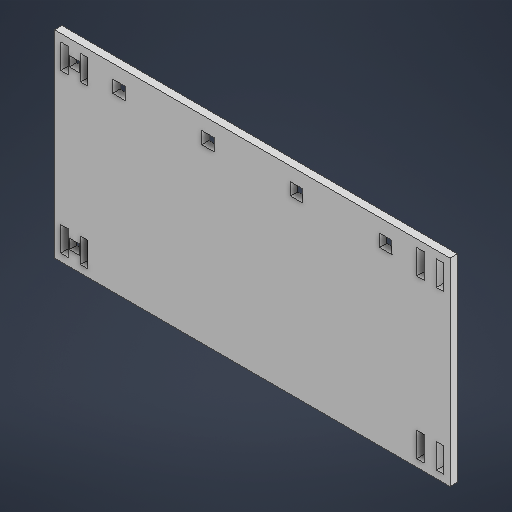
# Autodesk Inventor part: techo
Saved by Autodesk Inventor 2026 (Build 300175000, 175)
## iProperties
Created: 2026-05-15
Part Number: techo
Material: Generic
Document SubType Name: Modeling
Designer: juana
Density: 1 g/cm^3
Appearance: Default
Author: juana
Autodesk Inventor part; units mm, degrees
ref_plane "YZ Plane" through (0, 0, 0) normal (1, 0, 0) x (0, 1, 0)
ref_plane "XZ Plane" through (0, 0, 0) normal (0, 1, 0) x (-1, 0, 0)
ref_plane "XY Plane" through (0, 0, 0) normal (0, 0, 1) x (1, 0, 0)
sketch "Sketch1" plane through (0, 0, 0) normal (0, 0, 1) x (1, 0, 0)
  line L0 (0, 0) -> (160, 0)
  line L1 (160, 0) -> (160, 80)
  line L2 (160, 80) -> (0, 80)
  line L3 (0, 80) -> (0, 0)
  line L4 (2.5, 13) -> (5.5, 13)
  line L5 (5.5, 13) -> (5.5, 3)
  line L6 (5.5, 3) -> (2.5, 3)
  line L7 (2.5, 3) -> (2.5, 13)
  line L8 (10.5, 13) -> (13.5, 13)
  line L9 (13.5, 13) -> (13.5, 3)
  line L10 (13.5, 3) -> (10.5, 3)
  line L11 (10.5, 3) -> (10.5, 13)
  line L12 (0, 40) -> (160, 40) construction
  line L13 (80, 80) -> (80, 0) construction
  line L14 (0, 0) -> (0, 80)
  line L15 (2.5, 67) -> (5.5, 67)
  line L16 (5.5, 67) -> (5.5, 77)
  line L17 (5.5, 77) -> (2.5, 77)
  line L18 (2.5, 77) -> (2.5, 67)
  line L19 (10.5, 67) -> (13.5, 67)
  line L20 (13.5, 67) -> (13.5, 77)
  line L21 (13.5, 77) -> (10.5, 77)
  line L22 (10.5, 77) -> (10.5, 67)
  line L23 (157.5, 13) -> (154.5, 13)
  line L24 (154.5, 13) -> (154.5, 3)
  line L25 (154.5, 3) -> (157.5, 3)
  line L26 (157.5, 3) -> (157.5, 13)
  line L27 (149.5, 13) -> (146.5, 13)
  line L28 (146.5, 13) -> (146.5, 3)
  line L29 (146.5, 3) -> (149.5, 3)
  line L30 (149.5, 3) -> (149.5, 13)
  line L31 (154.5, 67) -> (154.5, 77)
  line L32 (157.5, 67) -> (154.5, 67)
  line L33 (157.5, 77) -> (157.5, 67)
  line L34 (146.5, 77) -> (149.5, 77)
  line L35 (149.5, 77) -> (149.5, 67)
  line L36 (149.5, 67) -> (146.5, 67)
  line L37 (146.5, 67) -> (146.5, 77)
  line L38 (154.5, 77) -> (157.5, 77)
  line L39 (2.5, 77) -> (157.5, 77) construction
  line L40 (157.5, 77) -> (157.5, 3) construction
  line L41 (157.5, 3) -> (2.5, 3) construction
  line L42 (2.5, 3) -> (2.5, 77) construction
  line L43 (6, 74) -> (10, 74)
  line L44 (10, 74) -> (10, 70)
  line L45 (10, 70) -> (6, 70)
  line L46 (6, 70) -> (6, 74)
  line L47 (5.5, 13) -> (5.5, 3)
  line L48 (6, 6) -> (10, 6)
  line L49 (10, 6) -> (10, 10)
  line L50 (10, 10) -> (6, 10)
  line L51 (6, 10) -> (6, 6)
  line L52 (23.49, 69.49) -> (28.51, 69.49)
  line L53 (28.51, 69.49) -> (28.51, 74.51)
  line L54 (28.51, 74.51) -> (23.49, 74.51)
  line L55 (23.49, 74.51) -> (23.49, 69.49)
  line L56 (59.49, 69.49) -> (64.51, 69.49)
  line L57 (64.51, 74.51) -> (59.49, 74.51)
  line L58 (64.51, 69.49) -> (64.51, 74.51)
  line L59 (59.49, 74.51) -> (59.49, 69.49)
  line L60 (95.49, 69.49) -> (100.51, 69.49)
  line L61 (100.51, 74.51) -> (95.49, 74.51)
  line L62 (100.51, 69.49) -> (100.51, 74.51)
  line L63 (95.49, 74.51) -> (95.49, 69.49)
  line L64 (131.49, 69.49) -> (136.51, 69.49)
  line L65 (136.51, 74.51) -> (131.49, 74.51)
  line L66 (136.51, 69.49) -> (136.51, 74.51)
  line L67 (131.49, 74.51) -> (131.49, 69.49)
  point P0 (23.49, 72)
  point P1 (10, 72)
  point P2 (26, 74.51)
  point P3 (62, 74.51)
  point P4 (59.49, 72)
  point P5 (98, 74.51)
  point P6 (95.49, 72)
  point P7 (134, 74.51)
  point P8 (131.49, 72)
  dimension "d0" = 80
  dimension "d1" = 160
  dimension "d2" = 3
  dimension "d3" = 2.5
  dimension "d4" = 3
  dimension "d5" = 10
  dimension "d6" = 5
  dimension "d7" = 3
  dimension "d8" = 0.5
  dimension "d9" = 0.5
  dimension "d10" = 3
  dimension "d11" = 5.02
  dimension "d12" = 5.02
  dimension "d13" = 23.5
  dimension "d16" = 36
  constraints: 136 end point, 30 symmetric about line, 12 parallel, 7 horizontal, 7 midpoint, 6 perpendicular, 2 equal length, 2 horizontal alignment, 30 other
  measures "d0" distance of L0.end L1.end
  measures "d1" distance of L0.start L0.end
  measures "d2" distance of L4.start L4.end
  measures "d3" distance between parallel lines of L3 L7
  measures "d4" distance between parallel lines of L0 L6
  measures "d5" distance of L4.end L5.end
  measures "d6" distance between parallel lines of L11 L5
  measures "d7" distance between parallel lines of L39 L43
  measures "d8" distance between parallel lines of L22 L44
  measures "d9" distance between parallel lines of L16 L46
  measures "d10" distance between parallel lines of L19 L45
  measures "d11" distance of L53.end L54.end
  measures "d12" distance of L52.end L53.end
  measures "d13" distance from line of L42 point (26, 74.51)
  measures "d16" distance of L52.end L56.end
extrude "Extrusion1" add sketch "Sketch1" along normal blind 3
body "Solid1"
